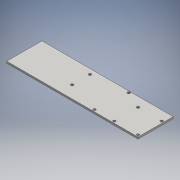
# Autodesk Inventor part: electronic_base
Saved by Autodesk Inventor 2016 (Build 200138000, 138)
## iProperties
Created: 2019-02-12
Part Number: electronic_base
Material: Generic
Document SubType Name: Modeling
Designer: LinJie
Density: 1 g/cm^3
Appearance: Default
Author: LinJie
Autodesk Inventor part; units mm, degrees
ref_plane "YZ Plane" through (0, 0, 0) normal (1, 0, 0) x (0, 1, 0)
ref_plane "XZ Plane" through (0, 0, 0) normal (0, 1, 0) x (-1, 0, 0)
ref_plane "XY Plane" through (0, 0, 0) normal (0, 0, 1) x (1, 0, 0)
sketch "Sketch1" plane through (0, 0, 0) normal (0, 0, 1) x (1, 0, 0)
  line L0 (-102.5, -27.5) -> (102.5, -27.5)
  line L1 (102.5, -27.5) -> (102.5, 27.5)
  line L2 (102.5, 27.5) -> (-102.5, 27.5)
  line L3 (-102.5, 27.5) -> (-102.5, -27.5)
  line L4 (-102.5, -27.5) -> (102.5, 27.5) construction
  line L5 (102.5, -27.5) -> (-102.5, 27.5) construction
  point P0 (0, 0)
  dimension "d0" = 205
  dimension "d1" = 55
  constraints: 12 end point, 2 midpoint, 2 parallel, 1 horizontal, 1 perpendicular
  measures "d0" distance of L2.end L1.end
  measures "d1" distance of L1.end L0.end
extrude "Extrusion1" add sketch "Sketch1" along normal blind 3
sketch "Sketch2" plane through (0, 0, 3) normal (0, 0, 1) x (1, 0, 0)
  line L0 (102.5, 27.5) -> (-102.5, 27.5) projected
  line L1 (-22.5, 27.5) -> (-22.5, -27.5) construction
  line L2 (-102.5, -27.5) -> (102.5, -27.5) projected
  line L3 (-102.5, 27.5) -> (-102.5, -27.5) projected
  line L4 (102.5, -27.5) -> (102.5, 27.5) projected
  point P0 (0, 0)
  point P1 (-19.5, 19.5)
  point P2 (-19.5, -8.5)
  point P3 (35.5, 25)
  point P4 (31.5, -24.5)
  point P5 (62.5, 12.5)
  point P6 (99.5, 12.5)
  point P7 (62.5, -24.5)
  point P8 (99.5, -24.5)
  dimension "d4" = 80
  dimension "d5" = 3
  dimension "d6" = 8
  dimension "d7" = 28
  dimension "d8" = 55
  dimension "d9" = 2.5
  dimension "d10" = 51
  dimension "d11" = 16
  dimension "d12" = 37
  dimension "d13" = 37
  dimension "d14" = 3
  dimension "d15" = 3
  constraints: 3 vertical alignment, 2 end point, 2 horizontal alignment, 2 point on line, 1 vertical
  measures "d4" distance between parallel lines of L3 L1
  measures "d5" distance from line of L1 point (-19.5, 19.5)
  measures "d6" distance from line of L0 point (-19.5, 19.5)
  measures "d7" distance of point (-19.5, 19.5) point (-19.5, -8.5)
  measures "d8" horizontal distance of point (-19.5, 19.5) point (35.5, 25)
  measures "d9" distance from line of L0 point (35.5, 25)
  measures "d10" horizontal distance of point (-19.5, -8.5) point (31.5, -24.5)
  measures "d11" vertical distance of point (31.5, -24.5) point (-19.5, -8.5)
  measures "d12" distance of point (99.5, 12.5) point (62.5, 12.5)
  measures "d13" distance of point (62.5, -24.5) point (62.5, 12.5)
  measures "d14" distance from line of L2 point (62.5, -24.5)
  measures "d15" distance from line of L4 point (99.5, -24.5)
hole "Hole1" at (-19.5, 19.5, 3) at (-19.5, -8.5, 3) at (35.5, 25, 3) at (31.5, -24.5, 3) at (62.5, 12.5, 3) at (99.5, 12.5, 3) at (62.5, -24.5, 3) at (99.5, -24.5, 3) direction (0, 0, -1) diameter 4 end through all
body "Solid1"
